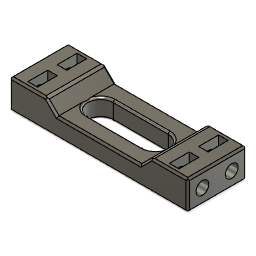
CoxaAssembly v6 (Autodesk Fusion 360 archive; units mm, degrees)
design "LegRib"
Autodesk Fusion 360 part; units mm, degrees
sketch "Sketch1" plane through (0, 0, 0) normal (0, 1, 0) x (1, 0, 0)
  line L0 (0, 0) -> (48.6, 0)
  line L1 (48.6, 0) -> (48.6, 16)
  line L2 (48.6, 16) -> (0, 16)
  line L3 (0, 16) -> (0, 0)
  dimension "d1" = 48.6
  dimension "d2" = 16
  constraint horizontal L0
  constraint vertical L1
  constraint horizontal L2
  constraint vertical L3
  constraint coincident L0.start L3.end
  measures "d1" distance of L1.end L2.end
  measures "d2" distance of L0.start L2.end
extrude "Extrude1" add sketch "Sketch1" along normal blind 8
sketch "Sketch2" plane through (0, 0, 0) normal (-1, 0, 0) x (0, 0, 1)
  line L0 (-16, 0) -> (0, 0)
  line L1 (0, 0) -> (0, 8)
  line L2 (0, 8) -> (-16, 8)
  line L3 (-16, 8) -> (-16, 0)
  line L4 (-16, 4) -> (0, 4) construction
  circle A0 centre (-12, 4) radius 1.75
  circle A1 centre (-4, 4) radius 1.75
  dimension "d5" = 3.5
  dimension "d6" = 3.5
  dimension "d7" = 16
  dimension "d8" = 4
  dimension "d9" = 4
  constraint midpoint L3 L4.start
  constraint midpoint L1 L4.end
  constraint coincident L4 A0.centre
  constraint coincident L4 A1.centre
  measures "d5" diameter of A0
  measures "d6" diameter of A1
  measures "d7" distance of L1.end L2.end
  measures "d8" distance of L3 A0.centre
  measures "d9" distance of L1 A1.centre
extrude "Extrude2" cut sketch "Sketch2" against normal blind 12 contours A0 | A1
ref_plane "WorkPlane1" through (5, 4, -8) normal (-1, 0, 0) x (0, 0, 1)
sketch "Sketch3" plane through (5, 4, -8) normal (-1, 0, 0) x (0, 0, -1)
  circle A0 centre (4, 0) radius 1.75
  circle A1 centre (-4, 0) radius 1.75
  line L0 (8, 4) -> (-8, 4)
  line L1 (-8, 4) -> (-8, -4)
  line L2 (-8, -4) -> (8, -4)
  line L3 (8, -4) -> (8, 4)
  line L4 (1.3, 1.5588) -> (1.3, -1.5588)
  line L5 (1.3, -1.5588) -> (4, -3.1177)
  line L6 (4, -3.1177) -> (6.7, -1.5588)
  line L7 (6.7, -1.5588) -> (6.7, 1.5588)
  line L8 (6.7, 1.5588) -> (4, 3.1177)
  line L9 (4, 3.1177) -> (1.3, 1.5588)
  line L10 (6.7, 4) -> (1.3, 4)
  line L11 (1.3, 4) -> (1.3, -4)
  line L12 (1.3, -4) -> (6.7, -4)
  line L13 (6.7, -4) -> (6.7, 4)
  point P0 (4, 0)
  dimension "d13" = 5.4
  constraint coincident P0 A0.centre
  constraint parallel L3 L7
  constraint horizontal L10
  constraint vertical L11
  constraint horizontal L12
  constraint vertical L13
  constraint coincident L2 L11.end
  constraint coincident L0 L10.start
  constraint collinear L7 L13
  constraint collinear L4 L11
  measures "d13" distance of L4 L7
extrude "Extrude3" cut sketch "Sketch3" along normal mid plane 2.6 contours L0 L8 L9 L10 L11 L13 | L4 L5 L6 L7 L8 L9 L11 L13 | L2 L5 L6 L11 L12 L13
ref_plane "WorkPlane2" through (24.3, 4, -8) normal (0, 0, -1) x (-1, 0, 0)
ref_plane "WorkPlane3" through (24.3, 4, -8) normal (-1, 0, 0) x (0, 0, 1)
mirror "Mirror1" about plane through (24.3, 4, -8) normal (0, 0, -1) of "Extrude3"
mirror "Mirror2" about plane through (24.3, 4, -8) normal (-1, 0, 0) of "Extrude2", "Extrude3", "Mirror1"
sketch "Sketch4" plane through (0, 0, 0) normal (0, 0, 1) x (1, 0, 0)
  line L0 (0, 0) -> (48.6, 0)
  line L1 (48.6, 0) -> (48.6, 8)
  line L2 (48.6, 8) -> (0, 8)
  line L3 (0, 8) -> (0, 0)
  line L4 (10, 8) -> (13, 5)
  line L5 (13, 5) -> (35.6, 5)
  line L6 (35.6, 5) -> (38.6, 8)
  dimension "d22" = 10
  dimension "d23" = 10
  dimension "d24" = 135
  dimension "d25" = 135
  dimension "d26" = 3
  constraint coincident L2 L4.start
  constraint parallel L2 L5
  constraint coincident L2 L6.end
  measures "d22" distance of L3 L4.start
  measures "d23" distance of L1 L6.end
  measures "d24" angle of L4 L5
  measures "d25" angle of L5 L6
  measures "d26" distance of L2 L5
extrude "Extrude4" cut sketch "Sketch4" against normal blind 16 contours L2 L4 L5 L6
sketch "Sketch5" plane through (0, 0, 0) normal (0, -1, 0) x (1, 0, 0)
  line L0 (42.3, -6.7) -> (42.3, -1.3)
  line L1 (42.3, -1.3) -> (44.9, -1.3)
  line L2 (44.9, -1.3) -> (44.9, -6.7)
  line L3 (44.9, -6.7) -> (42.3, -6.7)
  line L4 (42.3, -14.7) -> (42.3, -9.3)
  line L5 (42.3, -9.3) -> (44.9, -9.3)
  line L6 (44.9, -9.3) -> (44.9, -14.7)
  line L7 (44.9, -14.7) -> (42.3, -14.7)
  line L8 (6.3, -1.3) -> (6.3, -6.7)
  line L9 (6.3, -6.7) -> (3.7, -6.7)
  line L10 (3.7, -6.7) -> (3.7, -1.3)
  line L11 (3.7, -1.3) -> (6.3, -1.3)
  line L12 (6.3, -9.3) -> (6.3, -14.7)
  line L13 (6.3, -14.7) -> (3.7, -14.7)
  line L14 (3.7, -14.7) -> (3.7, -9.3)
  line L15 (3.7, -9.3) -> (6.3, -9.3)
  line L16 (0, 0) -> (0, -16)
  line L17 (0, -16) -> (48.6, -16)
  line L18 (48.6, -16) -> (48.6, 0)
  line L19 (48.6, 0) -> (0, 0)
  line L20 (0, -8) -> (48.6, -8) construction
  line L21 (16.8, -11.5) -> (31.8, -11.5)
  arc A0 (31.8, -11.5) -> (31.8, -4.5) centre (31.8, -8) ccw
  line L22 (31.8, -4.5) -> (16.8, -4.5)
  arc A1 (16.8, -4.5) -> (16.8, -11.5) centre (16.8, -8) ccw
  line L23 (16.8, -8) -> (31.8, -8) construction
  dimension "d29" = 7
  dimension "d30" = 15
  dimension "d31" = 48.6
  dimension "d32" = 16.8
  constraint midpoint L16 L20.start
  constraint midpoint L18 L20.end
  constraint tangent L21 A0
  constraint tangent A0 L22
  constraint parallel L21 L22
  constraint tangent L22 A1
  constraint tangent L21 A1
  constraint coincident L20 A0.centre
  constraint parallel L20 L23
  measures "d29" distance of L21 L22
  measures "d30" distance of A1.centre A0.centre
  measures "d31" distance of L16.start L18.end
  measures "d32" distance of L16 A1.centre
extrude "Extrude5" cut sketch "Sketch5" against normal up to surface (8 mm away) contours L21 A0 L22 A1
chamfer "Chamfer1" distance 0.5 angle 45 10 edges at (48.6, 8, -8) (5, 8, 0) (43.6, 8, 0) (0, 8, -8) (5, 8, -16) (43.6, 8, -16) (24.3, 0, -16) (48.6, 0, -8) (24.3, 0, 0) (0, 0, -8)
chamfer "Chamfer3" distance 0.5 angle 45 4 edges at (0, 4, -16) (0, 4, 0) (48.6, 4, 0) (48.6, 4, -16)
chamfer "Chamfer4" distance 0.5 angle 45 8 edges at (11.75, 6.25, 0) (24.3, 5, 0) (36.85, 6.25, 0) (38.6, 8, -8) (36.85, 6.25, -16) (24.3, 5, -16) (11.75, 6.25, -16) (10, 8, -8)
fillet "Fillet1" radius 0.5 4 edges at (13.3, 5, -8) (24.3, 5, -11.5) (35.3, 5, -8) (24.3, 5, -4.5)
fillet "Fillet2" radius 0.5 4 edges at (24.3, 0, -11.5) (13.3, 0, -8) (24.3, 0, -4.5) (35.3, 0, -8)
equation "d6 = d5"
equation "d8 = d7 / 4"
equation "d9 = d8"
equation "d23 = d22"
equation "d25 = d24"
equation "d32 = ( d31 - d30 ) / 2"
